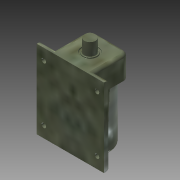
# Autodesk Inventor part: 砂轮电机
Saved by Autodesk Inventor 2015 (Build 190159000, 159)
## iProperties
Created: 2017-05-17
Part Number: 砂轮电机
Material: 常规
Document SubType Name: Modeling
Designer: Administrator
Density: 1 g/cm^3
Appearance: 预制平滑
Author: Administrator
Autodesk Inventor part; units mm, degrees
ref_plane "YZ Plane" through (0, 0, 0) normal (1, 0, 0) x (0, 1, 0)
ref_plane "XZ Plane" through (0, 0, 0) normal (0, 1, 0) x (-1, 0, 0)
sketch "草图1" plane through (0, 0, 0) normal (0, 0, 1) x (1, 0, 0)
  line L0 (-35, 70) -> (35, 70)
  line L1 (35, 70) -> (35, 0)
  line L2 (35, 0) -> (-35, 0)
  line L3 (-35, 0) -> (-35, 70)
  line L4 (-60, 8) -> (60, 8)
  line L5 (60, 8) -> (60, 0)
  line L6 (60, 0) -> (-60, 0)
  line L7 (-60, 0) -> (-60, 8)
  point P0 (0, 0)
  point P1 (0, 0)
  dimension "d0" = 70
  dimension "d1" = 8
  dimension "d2" = 120
  constraints: 16 end point, 4 parallel, 3 perpendicular, 2 horizontal, 2 midpoint, 1 coincident
  measures "d0" distance of L0.end L1.end
  measures "d1" distance of L4.end L5.end
  measures "d2" distance of L4.start L4.end
extrude "拉伸1" add sketch "草图1" along normal blind 140
sketch "草图2" plane through (0, 0, 0) normal (0, 0, -1) x (-1, 0, 0)
  circle A0 centre (0, 35) radius 35
  line L0 (-35, 8) -> (-35, 70) projected
  line L1 (-35, 70) -> (35, 70) projected
  line L2 (-22.2711, 8) -> (-35, 8)
  line L3 (-35, 70) -> (0, 70)
  line L4 (-35, 70) -> (35, 70) projected
  line L5 (35, 70) -> (35, 8)
  line L6 (35, 70) -> (35, 8) projected
  line L7 (35, 8) -> (22.2711, 8)
  point P0 (0, 0)
  dimension "d5" = 70
  constraints: 8 end point, 2 point on circle, 2 tangent, 1 centre point, 1 collinear, 1 horizontal, 1 midpoint, 1 point on line
  measures "d5" diameter of A0
extrude "拉伸2" cut sketch "草图2" against normal blind 100 contours L5 L7 A0 | A0 L1 L5 | A0 L0 L1 | A0 L2 L0
fillet "圆角1" radius 10 2 edges at (35, 70, 120) (-35, 70, 120)
fillet "圆角2" radius 5.5 2 edges at (22.2711, 8, 50) (-22.2711, 8, 50)
fillet "圆角3" radius 5 5 edges at (29.5101, 10.8362, 0) (0, 70, 0) (-29.5101, 10.8362, 0) (-47.161, 8, 0) (47.161, 8, 0)
fillet "圆角4" radius 5 7 edges at (-32.0711, 67.0711, 140) (0, 70, 140) (32.0711, 67.0711, 140) (35, 34, 140) (-35, 34, 140) (-47.5, 8, 140) (47.5, 8, 140)
sketch "草图3" plane through (0, 0, 140) normal (0, 0, 1) x (1, 0, 0)
  circle A0 centre (0, 35) radius 10
  arc A1 (35, 35) -> (0, 70) centre (0, 35) ccw projected
  point P0 (0, 0)
  dimension "d12" = 20
  constraints: 1 centre point, 1 concentric
  measures "d12" diameter of A0
extrude "拉伸3" add sketch "草图3" along normal blind 22
sketch "草图4" plane through (0, 0, 140) normal (0, 0, 1) x (1, 0, 0)
  circle A0 centre (0, 35) radius 10.5
  circle A1 centre (0, 35) radius 10
  circle A2 centre (0, 35) radius 10 projected
  circle A3 centre (0, 35) radius 12.5
  circle A4 centre (0, 35) radius 15
  point P0 (0, 0)
  dimension "d15" = 21
  dimension "d16" = 20
  dimension "d17" = 25
  dimension "d18" = 30
  constraints: 4 centre point, 3 concentric, 2 coincident
  measures "d15" diameter of A0
  measures "d16" diameter of A1
  measures "d17" diameter of A3
  measures "d18" diameter of A4
extrude "拉伸4" cut sketch "草图4" against normal blind 2
fillet "圆角5" radius 0.5 4 edges at (-15, 35, 140) (-15, 35, 138) (-12.5, 35, 140) (-12.5, 35, 138)
sketch "草图5" plane through (34.322, 8, 5) normal (0, 1, 0) x (1, 0, 0)
  circle A0 centre (13.178, -15) radius 4
  circle A1 centre (13.178, -115) radius 4
  circle A2 centre (-81.822, -15) radius 4
  circle A3 centre (-81.822, -115) radius 4
  line L0 (25.678, 0) -> (25.678, -130) projected
  line L1 (-94.322, 5) -> (-94.322, -135) projected
  line L2 (-4.322, -135) -> (25.678, -135) projected
  line L3 (-94.322, -135) -> (-64.322, -135) projected
  line L4 (25.678, 5) -> (0, 5) projected
  line L5 (-68.644, 5) -> (-94.322, 5) projected
  point P0 (-34.322, 5)
  dimension "d22" = 8
  dimension "d23" = 8
  dimension "d24" = 8
  dimension "d25" = 8
  dimension "d26" = 12.5
  dimension "d27" = 12.5
  dimension "d28" = 12.5
  dimension "d29" = 12.5
  dimension "d30" = 20
  dimension "d31" = 20
  dimension "d32" = 20
  dimension "d33" = 20
  constraints: 4 centre point
  measures "d22" diameter of A0
  measures "d23" diameter of A1
  measures "d24" diameter of A2
  measures "d25" diameter of A3
  measures "d26" distance from line of L0 A0.centre
  measures "d27" distance from line of L0 A1.centre
  measures "d28" distance from line of L1 A2.centre
  measures "d29" distance from line of L1 A3.centre
  measures "d30" distance from line of L2 A1.centre
  measures "d31" distance from line of L3 A3.centre
  measures "d32" distance from line of L4 A0.centre
  measures "d33" distance from line of L5 A2.centre
extrude "拉伸5" cut sketch "草图5" against normal through all
ref_plane "工作平面1" through (0, 45, 140) normal (0, -1, 0) x (1, 0, 0)
sketch "草图6" plane through (0, 45, 140) normal (0, -1, 0) x (1, 0, 0)
  circle A0 centre (0, 12) radius 2
  line L0 (10, 22) -> (-10, 22) projected
  line L1 (0, -140) -> (0, -150.2125)
  dimension "d36" = 4
  dimension "d37" = 10
  dimension "d38" = 10.2125
  constraints: 2 end point, 1 centre point, 1 point on line, 1 vertical
  measures "d36" diameter of A0
  measures "d37" distance from line of L0 A0.centre
  measures "d38" distance of L1.start L1.end
extrude "拉伸6" cut sketch "草图6" along normal blind 2
